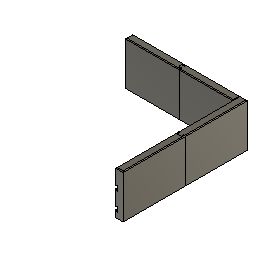
ShelfOrganizer (Autodesk Fusion 360 design; units mm, degrees)
part number: 2026-05-06-18-24-14-128
Autodesk Fusion 360 part; units mm, degrees
sketch "Sketch1" plane through (0, 0, 0) normal (0, 0, 1) x (1, 0, 0)
  line L0 (0, 0) -> (20, 0)
  line L1 (20, 0) -> (20, 342)
  line L2 (20, 342) -> (0, 342)
  line L3 (0, 342) -> (0, 0)
  line L4 (15, 171) -> (17, 165)
  line L5 (17, 165) -> (3, 165)
  line L6 (3, 165) -> (5, 171)
  line L7 (20, 171) -> (15, 171)
  line L8 (5, 171) -> (0, 171)
  dimension "d1" = 20
  dimension "d2" = 342
  dimension "d13" = 171
  constraint horizontal L0
  constraint vertical L1
  constraint horizontal L2
  constraint vertical L3
  constraint coincident L0.start L3.end
  constraint coincident L1 L7.start
  constraint coincident L3 L8.end
  constraint perpendicular L3 L8
  constraint parallel L5 L7
  constraint collinear L7 L8
  measures "d1" distance of L0.start L0.end
  measures "d2" distance of L0.start L2.end
  measures "d13" distance of L0.start L8.end
extrude "Extrude4" add sketch "Sketch1" along normal blind 120 contours L1 L2 L3 L4 L5 L6 L7 L8 makes body 1
extrude "Extrude5" add sketch "Sketch1" along normal blind 120 separate body contours L0 L1 L3 L4 L5 L6 L7 L8 makes body 2
sketch "Sketch4" plane through (0, 342, 0) normal (0, 1, 0) x (-1, 0, 0)
  line L0 (-20, 0) -> (0, 0)
  line L1 (0, 0) -> (0, 120)
  line L2 (0, 120) -> (-20, 120)
  line L3 (-20, 120) -> (-20, 0)
  line L4 (0, 25) -> (-5, 30)
  line L5 (-5, 30) -> (-5, 15)
  line L6 (-5, 15) -> (0, 20)
  line L7 (0, 75) -> (-5, 80)
  line L8 (-5, 80) -> (-5, 65)
  line L9 (-5, 65) -> (0, 70)
  line L10 (-5, 0) -> (295, 0)
  line L11 (295, 0) -> (295, 120)
  line L12 (295, 120) -> (-5, 120)
  line L13 (-5, 120) -> (-5, 0)
  dimension "d18" = 20
  dimension "d19" = 45
  dimension "d20" = 300
  dimension "d21" = 120
  constraint coincident L1 L4.start
  constraint parallel L1 L5
  constraint coincident L1 L6.end
  constraint perpendicular L4 L6
  constraint perpendicular L7 L9
  constraint horizontal L10
  constraint vertical L11
  constraint horizontal L12
  constraint vertical L13
  constraint coincident L0 L10.start
  measures "d18" distance of L0.end L6.end
  measures "d19" distance of L4.start L9.end
  measures "d20" distance of L10.start L10.end
  measures "d21" distance of L10.start L12.end
extrude "Extrude6" cut sketch "Sketch4" along normal through all and the other way through all contours L1 L4 L5 L6 L13 | L1 L7 L8 L9 L13 bodies 1 2
extrude "Extrude7" add sketch "Sketch4" against normal blind 20 separate body contours L1 L10 L11 L12 | L1 L4 L5 L6 L13 | L1 L7 L8 L9 L13 makes body 3
move_face "OffsetFaces1" offset -0.3 5 faces at (13, 165, 66.6667) (15.6667, 169, 40) (3.6667, 167, 92.6667) (3.6667, 167, 53.3333) (3.6667, 167, 10.6667) on bodies 2
move_face "OffsetFaces2" offset -0.3 6 faces at (2.5279, 54.9, 77.5279) (2.5279, 54.9, 67.4721) (2.5279, 54.9, 17.4721) (2.5279, 54.9, 27.5279) (5, 54.9, 25) (5, 54.9, 75) on bodies 2
move_face "OffsetFaces3" offset -0.3 6 faces at (1.6667, 228, 76.6667) (1.6667, 228, 26.6667) (5, 228, 25) (5, 228, 75) (1.6667, 228, 18.3333) (1.6667, 228, 68.3333) on bodies 1
move_face "OffsetFaces4" offset -0.2 4 faces at (18.3333, 171, 40) (1.6667, 171, 91.9495) (1.6667, 171, 53.1919) (1.6667, 171, 11.3838) on bodies 1
move_face "OffsetFaces5" offset -0.2 3 faces at (0, 335.3333, 90) (0, 328.6667, 40) (0, 335.3333, 6.6667) on bodies 3
ref_plane "WorkPlane2" through (-147.6, 332, 60) normal (-1, 0, 0) x (0, 0, -1)
sketch "Sketch6" plane through (0, 0, 120) normal (0, 0, 1) x (-1, 0, 0)
  line L0 (0.2, -342) -> (295, -342)
  line L1 (295, -342) -> (295, -322)
  line L2 (295, -322) -> (0.2, -322)
  line L3 (0.2, -322) -> (0.2, -342)
  circle A0 centre (150.6, -332) radius 5.053
  line L4 (147.6, -281.1526) -> (147.6, -382.8474)
  dimension "d33" = 3
  measures "d33" distance of A0.centre L4
split "Split2" by plane through (-147.6, 332, 60) normal (-1, 0, 0) bodies 3 makes body 4 at (-196.7333, 342, 80)
extrude "Extrude8" add sketch "Sketch6" against normal blind 120 contours A0 L4 picked at (150.123, -331.2806) bodies 3
extrude "Extrude9" cut sketch "Sketch6" against normal blind 120 contours A0 L4 picked at (150.123, -331.2806) bodies 4
move_face "OffsetFaces8" offset -0.2 3 faces at (-147.6, 340.022, 40) (-153.6143, 336.0555, 40) (-147.6, 325.956, 40) on bodies 3
fillet "Fillet2" radius 2 11 edges at (20, 256.6, 120) (10, 342, 120) (0, 256.6, 120) (0, 85.5, 120) (20, 85.5, 120) (10, 0, 120) (-73.8, 322, 120) (-73.8, 342, 120) (-221.3, 342, 120) (-221.3, 322, 120) (-295, 332, 120) on bodies 1 2 3 4
equation "d13 = ( 342 / 2 ) * 1 mm"
named bodies: "CrossBar1", "CrossBar2", "LongBar", "LongBar (1)"
